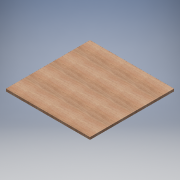
# Autodesk Inventor part: Desk
Saved by Autodesk Inventor 2018 (Build 220112000, 112)
## iProperties
Created: 2018-02-10
Part Number: Desk
Material: Wood (Birch)
Document SubType Name: Modeling
Designer: ConnorDevitt
Density: 0.55 g/cm^3
Appearance: Birch - Natural Polished
Author: ConnorDevitt
Autodesk Inventor part; units mm, degrees
ref_plane "YZ Plane" through (0, 0, 0) normal (1, 0, 0) x (0, 1, 0)
ref_plane "XZ Plane" through (0, 0, 0) normal (0, 1, 0) x (-1, 0, 0)
ref_plane "XY Plane" through (0, 0, 0) normal (0, 0, 1) x (1, 0, 0)
sketch "Sketch1" plane through (0, 0, 0) normal (0, 1, 0) x (-1, 0, 0)
  line L0 (-444.5, 444.5) -> (444.5, 444.5)
  line L1 (444.5, 444.5) -> (444.5, -444.5)
  line L2 (444.5, -444.5) -> (-444.5, -444.5)
  line L3 (-444.5, -444.5) -> (-444.5, 444.5)
  line L4 (-444.5, 444.5) -> (444.5, -444.5) construction
  line L5 (444.5, 444.5) -> (-444.5, -444.5) construction
  point P0 (0, 0)
  dimension "d0" = 889
  dimension "d1" = 889
  constraints: 12 end point, 2 midpoint, 2 parallel, 1 horizontal, 1 perpendicular
  measures "d0" distance of L0.end L1.end
  measures "d1" distance of L1.end L2.end
extrude "Extrusion1" add sketch "Sketch1" along normal blind 25.4
body "Solid1"
